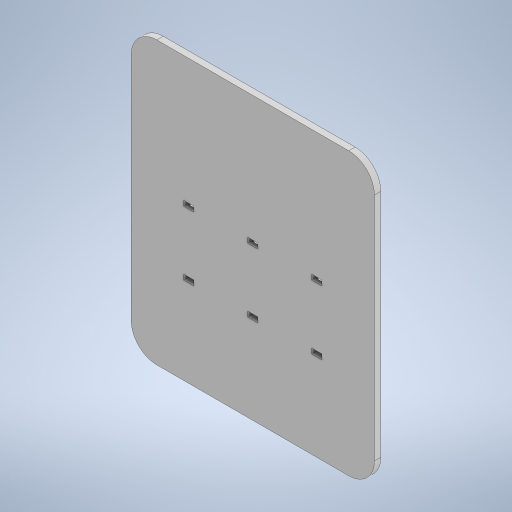
# Autodesk Inventor part: Plate_mount
Saved by Autodesk Inventor 2023 (Build 270158000, 158)
## iProperties
Created: 2022-11-05
Part Number: Plate_mount
Material: Generisch
Document SubType Name: Modeling
Designer: RubenStein
Density: 1 g/cm^3
Appearance: Vorgabe
Author: RubenStein
Autodesk Inventor part; units mm, degrees
ref_plane "YZ Plane" through (0, 0, 0) normal (1, 0, 0) x (0, 1, 0)
ref_plane "XZ Plane" through (0, 0, 0) normal (0, 1, 0) x (-1, 0, 0)
ref_plane "XY Plane" through (0, 0, 0) normal (0, 0, 1) x (1, 0, 0)
sketch "Skizze1" plane through (0, 0, 0) normal (0, 0, 1) x (1, 0, 0)
  line L0 (0, 0) -> (190, 0)
  line L1 (190, 0) -> (190, 220)
  line L2 (190, 220) -> (0, 220)
  line L3 (0, 220) -> (0, 0)
  dimension "d0" = 190
  dimension "d19" = 220
  constraints: 8 end point, 2 parallel, 1 horizontal, 1 perpendicular
  measures "d0" distance of L1.end L2.end
  measures "d19" distance of L0.end L1.end
extrude "Extrusion1" add sketch "Skizze1" along normal blind 5
fillet "Rundung1" radius 20 4 edges at (190, 220, 2.5) (0, 220, 2.5) (190, 0, 2.5) (0, 0, 2.5)
sketch "Skizze2" plane through (0, 0, 5) normal (0, 0, 1) x (1, 0, 0)
  line L0 (20, 170) -> (170, 170) construction
  line L1 (170, 170) -> (170, 20) construction
  line L2 (170, 20) -> (20, 20) construction
  line L3 (20, 20) -> (20, 170) construction
  line L4 (0, 200) -> (0, 20) construction
  line L5 (20, 0) -> (170, 0) construction
  line L6 (70, 170) -> (70, 20) construction
  line L7 (120, 170) -> (120, 20) construction
  line L8 (20, 120) -> (170, 120) construction
  line L9 (20, 70) -> (170, 70) construction
  line L10 (49, 118) -> (41, 118)
  line L11 (41, 118) -> (41, 122)
  line L12 (41, 122) -> (49, 122)
  line L13 (49, 122) -> (49, 118)
  line L14 (49, 118) -> (41, 122) construction
  line L15 (41, 118) -> (49, 122) construction
  line L16 (99, 118) -> (91, 118)
  line L17 (91, 118) -> (91, 122)
  line L18 (91, 122) -> (99, 122)
  line L19 (99, 122) -> (99, 118)
  line L20 (99, 118) -> (91, 122) construction
  line L21 (91, 118) -> (99, 122) construction
  line L22 (149, 118) -> (141, 118)
  line L23 (141, 118) -> (141, 122)
  line L24 (141, 122) -> (149, 122)
  line L25 (149, 122) -> (149, 118)
  line L26 (149, 118) -> (141, 122) construction
  line L27 (141, 118) -> (149, 122) construction
  line L28 (149, 68) -> (141, 68)
  line L29 (141, 68) -> (141, 72)
  line L30 (141, 72) -> (149, 72)
  line L31 (149, 72) -> (149, 68)
  line L32 (149, 68) -> (141, 72) construction
  line L33 (141, 68) -> (149, 72) construction
  line L34 (49, 68) -> (41, 68)
  line L35 (41, 68) -> (41, 72)
  line L36 (41, 72) -> (49, 72)
  line L37 (49, 72) -> (49, 68)
  line L38 (49, 68) -> (41, 72) construction
  line L39 (41, 68) -> (49, 72) construction
  line L40 (99, 68) -> (91, 68)
  line L41 (91, 68) -> (91, 72)
  line L42 (91, 72) -> (99, 72)
  line L43 (99, 72) -> (99, 68)
  line L44 (99, 68) -> (91, 72) construction
  line L45 (91, 68) -> (99, 72) construction
  point P0 (0, 0)
  point P1 (45, 120)
  point P2 (95, 120)
  point P3 (145, 120)
  point P4 (145, 70)
  point P5 (45, 70)
  point P6 (95, 70)
  dimension "d4" = 150
  dimension "d5" = 20
  dimension "d6" = 20
  dimension "d7" = 50
  dimension "d8" = 50
  dimension "d9" = 50
  dimension "d10" = 50
  dimension "d11" = 8
  dimension "d12" = 4
  dimension "d13" = 50
  dimension "d14" = 50
  dimension "d15" = 50
  dimension "d16" = 50
  constraints: 88 end point, 14 midpoint, 14 parallel, 14 point on line, 11 perpendicular, 9 equal length, 7 horizontal
  measures "d4" distance of L0.start L0.end
  measures "d5" distance between parallel lines of L4 L3
  measures "d6" distance between parallel lines of L5 L2
  measures "d7" distance between parallel lines of L3 L6
  measures "d8" distance between parallel lines of L2 L9
  measures "d9" distance between parallel lines of L8 L9
  measures "d10" distance between parallel lines of L7 L6
  measures "d11" distance of L11.end L12.end
  measures "d12" distance of L10.end L11.end
  measures "d13" distance of point (95, 120) point (45, 120)
  measures "d14" distance of point (145, 120) point (95, 120)
  measures "d15" distance of point (95, 70) point (45, 70)
  measures "d16" distance of point (145, 70) point (95, 70)
extrude "Extrusion2" cut sketch "Skizze2" against normal through all
sketch "Skizze3" plane through (0, 0, 0) normal (0, 0, -1) x (-1, 0, 0)
  line L0 (-41, 68) -> (-41, 72) projected
  line L1 (-41, 68) -> (-49, 68)
  line L2 (-49, 68) -> (-49, 210)
  line L3 (-49, 210) -> (-41, 210)
  line L4 (-41, 210) -> (-41, 68)
  line L5 (-99, 68) -> (-91, 68) projected
  line L6 (-91, 68) -> (-99, 68)
  line L7 (-99, 68) -> (-99, 210)
  line L8 (-99, 210) -> (-91, 210)
  line L9 (-91, 210) -> (-91, 68)
  line L10 (-141, 68) -> (-149, 68) projected
  line L11 (-141, 68) -> (-149, 68)
  line L12 (-149, 68) -> (-149, 210)
  line L13 (-149, 210) -> (-141, 210)
  line L14 (-141, 210) -> (-141, 68)
  line L15 (-49, 68) -> (-49, 72) projected
  line L16 (-170, 220) -> (-20, 220) projected
  point P0 (0, 0)
  dimension "d20" = 10
  constraints: 24 end point, 6 parallel, 3 equal length, 3 horizontal, 3 perpendicular, 1 collinear, 1 point on line
  measures "d20" distance between parallel lines of L16 L3
extrude "Extrusion3" cut sketch "Skizze3" against normal blind 2
equation "\"d6\" = d5"
equation "\"d8\" = d7"
equation "\"d9\" = d7"
equation "\"d10\" = d7"
equation "\"d14\" = d13"
equation "\"d15\" = d13"
equation "\"d16\" = d13"
